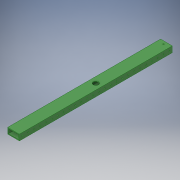
# Autodesk Inventor part: kermit frame 8
Saved by Autodesk Inventor 2018.2 (Build 222227000, 227)
## iProperties
Created: 2018-02-03
Part Number: kermit frame 8
Material: Generic
Document SubType Name: Modeling
Designer: cruz.anthony
Density: 1 g/cm^3
Appearance: Smooth - Dark Forest Green
Author: cruz.anthony
Autodesk Inventor part; units mm, degrees
ref_plane "YZ Plane" through (0, 0, 0) normal (1, 0, 0) x (0, 1, 0)
ref_plane "XZ Plane" through (0, 0, 0) normal (0, 1, 0) x (-1, 0, 0)
ref_plane "XY Plane" through (0, 0, 0) normal (0, 0, 1) x (1, 0, 0)
sketch "Sketch1" plane through (0, 0, 0) normal (0, 1, 0) x (-1, 0, 0)
  line L0 (0, 0) -> (50.8, 0)
  line L1 (50.8, 0) -> (50.8, -660.4)
  line L2 (50.8, -660.4) -> (0, -660.4)
  line L3 (0, -660.4) -> (0, 0)
  dimension "d0" = 50.8
  dimension "d1" = 660.4
  constraints: 8 end point, 2 parallel, 1 horizontal, 1 perpendicular
  measures "d0" distance of L1.end L2.end
  measures "d1" distance of L0.end L1.end
extrude "Extrusion1" add sketch "Sketch1" along normal blind 25.4
sketch "Sketch3" plane through (-50.8, 0, 0) normal (0, 0, 1) x (1, 0, 0)
  line L0 (3.175, 22.225) -> (47.625, 22.225)
  line L1 (47.625, 22.225) -> (47.625, 3.175)
  line L2 (47.625, 3.175) -> (3.175, 3.175)
  line L3 (3.175, 3.175) -> (3.175, 22.225)
  line L4 (0, 25.4) -> (50.8, 25.4) projected
  line L5 (0, 0) -> (0, 25.4) projected
  line L6 (50.8, 0) -> (0, 0) projected
  line L7 (50.8, 0) -> (50.8, 25.4) projected
  dimension "d16" = 3.175
  dimension "d17" = 3.175
  dimension "d18" = 3.175
  dimension "d19" = 3.175
  constraints: 8 end point, 2 parallel, 1 horizontal, 1 perpendicular
  measures "d16" distance between parallel lines of L4 L0
  measures "d17" distance between parallel lines of L5 L3
  measures "d18" distance between parallel lines of L6 L2
  measures "d19" distance between parallel lines of L7 L1
extrude "Extrusion3" cut sketch "Sketch3" against normal blind 660.4 contours L0 L1 L2 L3
sketch "Sketch4" plane through (0, 0, 0) normal (1, 0, 0) x (0, 0, -1)
  circle A0 centre (12.7, 12.7) radius 1.9685
  line L0 (0, 25.4) -> (660.4, 25.4) projected
  line L1 (0, 0) -> (0, 25.4) projected
  circle A1 centre (38.1, 12.7) radius 1.9685
  circle A2 centre (63.5, 12.7) radius 1.9685
  circle A3 centre (88.9, 12.7) radius 1.9685
  circle A4 centre (114.3, 12.7) radius 1.9685
  circle A5 centre (139.7, 12.7) radius 1.9685
  circle A6 centre (165.1, 12.7) radius 1.9685
  circle A7 centre (190.5, 12.7) radius 1.9685
  circle A8 centre (215.9, 12.7) radius 1.9685
  circle A9 centre (241.3, 12.7) radius 1.9685
  circle A10 centre (266.7, 12.7) radius 1.9685
  circle A11 centre (292.1, 12.7) radius 1.9685
  circle A12 centre (317.5, 12.7) radius 1.9685
  circle A13 centre (342.9, 12.7) radius 1.9685
  circle A14 centre (368.3, 12.7) radius 1.9685
  circle A15 centre (393.7, 12.7) radius 1.9685
  circle A16 centre (419.1, 12.7) radius 1.9685
  circle A17 centre (444.5, 12.7) radius 1.9685
  circle A18 centre (469.9, 12.7) radius 1.9685
  circle A19 centre (495.3, 12.7) radius 1.9685
  circle A20 centre (520.7, 12.7) radius 1.9685
  circle A21 centre (546.1, 12.7) radius 1.9685
  circle A22 centre (571.5, 12.7) radius 1.9685
  circle A23 centre (596.9, 12.7) radius 1.9685
  circle A24 centre (622.3, 12.7) radius 1.9685
  circle A25 centre (647.7, 12.7) radius 1.9685
  dimension "d22" = 3.937
  dimension "d23" = 12.7
  dimension "d24" = 12.7
  dimension "d27" = 25.4
  constraints: 26 centre point, 1 horizontal, 50 other
  measures "d22" diameter of A0
  measures "d23" distance from line of L0 A0.centre
  measures "d24" distance from line of L1 A0.centre
  measures "d27" distance of A0.centre A1.centre
extrude "Extrusion4" cut sketch "Sketch4" against normal blind 50.8
sketch "Sketch5" plane through (0, 25.4, 0) normal (0, 1, 0) x (1, 0, 0)
  circle A0 centre (-25.4, 355.6) radius 11.43
  line L0 (-50.8, 660.4) -> (-50.8, 0) projected
  circle A1 centre (-25.4, 647.7) radius 2.54
  line L1 (0, 660.4) -> (-50.8, 660.4) projected
  point P0 (0, 0)
  dimension "d34" = 22.86
  dimension "d35" = 25.4
  dimension "d36" = 304.8
  dimension "d39" = 5.08
  dimension "d40" = 25.4
  dimension "d41" = 12.7
  constraints: 2 centre point
  measures "d34" diameter of A0
  measures "d35" distance from line of L0 A0.centre
  measures "d36" vertical distance of L0.start A0.centre
  measures "d39" diameter of A1
  measures "d40" distance from line of L0 A1.centre
  measures "d41" distance from line of L1 A1.centre
extrude "Extrusion5" cut sketch "Sketch5" against normal blind 25.4
body "Solid1"
